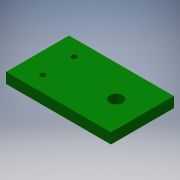
# Autodesk Inventor part: top bracket
Saved by Autodesk Inventor 2017 SP1 (Build 210196100, 196)
## iProperties
Created: 2018-01-25
Part Number: top bracket
Material: Generic
Document SubType Name: Modeling
Designer: Ben
Density: 1 g/cm^3
Appearance: Dark Green
Author: Ben
Autodesk Inventor part; units mm, degrees
ref_plane "YZ Plane" through (0, 0, 0) normal (1, 0, 0) x (0, 1, 0)
ref_plane "XZ Plane" through (0, 0, 0) normal (0, 1, 0) x (-1, 0, 0)
ref_plane "XY Plane" through (0, 0, 0) normal (0, 0, 1) x (1, 0, 0)
sketch "Sketch1" plane through (0, 0, 0) normal (0, 1, 0) x (-1, 0, 0)
  line L0 (-31.75, 19.05) -> (31.75, 19.05)
  line L1 (31.75, 19.05) -> (31.75, -19.05)
  line L2 (31.75, -19.05) -> (-31.75, -19.05)
  line L3 (-31.75, -19.05) -> (-31.75, 19.05)
  line L4 (-31.75, 19.05) -> (31.75, -19.05) construction
  line L5 (31.75, 19.05) -> (-31.75, -19.05) construction
  line L6 (6.35, -19.05) -> (6.35, 19.05) construction
  line L7 (31.75, 0) -> (-31.75, 0) construction
  circle A0 centre (-15.875, 0) radius 3.9688
  line L8 (19.05, -19.05) -> (19.05, 0) construction
  line L9 (19.05, 0) -> (19.05, 19.05) construction
  circle A1 centre (19.05, -9.525) radius 1.5875
  circle A2 centre (19.05, 9.525) radius 1.5875
  point P0 (0, 0)
  dimension "d0" = 63.5
  dimension "d1" = 38.1
  dimension "d2" = 25.4
  dimension "d3" = 7.9375
  dimension "d4" = 22.225
  dimension "d7" = 12.7
  dimension "d8" = 3.175
  constraints: 20 end point, 6 midpoint, 6 point on line, 4 perpendicular, 3 centre point, 2 parallel, 1 equal radius, 1 horizontal
  measures "d0" distance of L1.end L2.end
  measures "d1" distance of L0.end L1.end
  measures "d2" distance between parallel lines of L1 L6
  measures "d3" diameter of A0
  measures "d4" distance from line of L6 A0.centre
  measures "d7" distance between parallel lines of L6 L8
  measures "d8" diameter of A1
extrude "Extrusion1" add sketch "Sketch1" along normal blind 6.35
body "Solid1"
